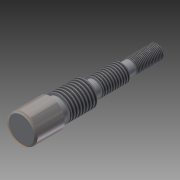
# Autodesk Inventor part: 13_3
Saved by Autodesk Inventor 2015 (Build 190159000, 159)
## iProperties
Created: 2015-03-30
Part Number: 13_3
Material: Generic
Document SubType Name: Modeling
Designer: WASHHSST
Density: 1 g/cm^3
Appearance: Default
Author: WASHHSST
Autodesk Inventor part; units mm, degrees
ref_plane "YZ Plane" through (0, 0, 0) normal (1, 0, 0) x (0, 1, 0)
ref_plane "XZ Plane" through (0, 0, 0) normal (0, 1, 0) x (-1, 0, 0)
ref_plane "XY Plane" through (0, 0, 0) normal (0, 0, 1) x (1, 0, 0)
sketch "Sketch2" plane through (0, 0, 0) normal (0, 0, 1) x (1, 0, 0)
  circle A0 centre (0, 0) radius 12.7
  dimension "d4" = 25.4
  constraints: 1 centre point, 1 coincident
  measures "d4" diameter of A0
extrude "Extrusion2" add sketch "Sketch2" against normal blind 25.4
chamfer "Chamfer1" distance 1.524 angle 45 1 edges at (-12.7, 0, 0) measured on face at (-12.2, 0, 0)
sketch "Sketch3" plane through (0, 0, -25.4) normal (0, 0, -1) x (-1, 0, 0)
  circle A0 centre (0, 0) radius 9.144
  dimension "d10" = 18.288
  constraints: 1 centre point, 1 coincident
  measures "d10" diameter of A0
extrude "Extrusion3" add sketch "Sketch3" along normal blind 6.35
sketch "Sketch4" plane through (0, 0, -31.75) normal (0, 0, -1) x (-1, 0, 0)
  circle A0 centre (0, 0) radius 11.049
  dimension "d13" = 22.098
  constraints: 1 centre point, 1 coincident
  measures "d13" diameter of A0
extrude "Extrusion4" add sketch "Sketch4" along normal blind 25.4
thread "Thread1" size "7/8-9 UNC" class "2A" standard "ANSI Unified Screw Threads" full length
chamfer "Chamfer2" distance 1.524 angle 45 1 edges at (11.049, 0, -57.15) measured on face at (10.549, 0, -57.15)
sketch "Sketch5" plane through (0, 0, -57.15) normal (0, 0, -1) x (-1, 0, 0)
  circle A0 centre (0, 0) radius 6.477
  dimension "d21" = 12.954
  constraints: 1 centre point, 1 coincident
  measures "d21" diameter of A0
extrude "Extrusion5" add sketch "Sketch5" along normal blind 6.35
sketch "Sketch6" plane through (0, 0, -63.5) normal (0, 0, -1) x (-1, 0, 0)
  circle A0 centre (0, 0) radius 7.874
  dimension "d24" = 15.748
  constraints: 1 centre point, 1 coincident
  measures "d24" diameter of A0
extrude "Extrusion6" add sketch "Sketch6" along normal blind 25.4
thread "Thread2" size "5/8-11 UNC" class "2A" standard "ANSI Unified Screw Threads" full length
chamfer "Chamfer3" distance 1.524 angle 45 1 edges at (7.874, 0, -88.9) measured on face at (7.374, 0, -88.9)
sketch "Sketch7" plane through (0, 0, -88.9) normal (0, 0, -1) x (-1, 0, 0)
  circle A0 centre (0, 0) radius 5.461
  dimension "d32" = 10.922
  constraints: 1 centre point, 1 coincident
  measures "d32" diameter of A0
extrude "Extrusion7" add sketch "Sketch7" along normal blind 6.35
sketch "Sketch8" plane through (0, 0, -95.25) normal (0, 0, -1) x (-1, 0, 0)
  circle A0 centre (0, 0) radius 6.35
  dimension "d35" = 12.7
  constraints: 1 centre point, 1 coincident
  measures "d35" diameter of A0
extrude "Extrusion8" add sketch "Sketch8" along normal blind 25.4
thread "Thread3" size "1/2-20 UNF" class "2A" standard "ANSI Unified Screw Threads" full length
chamfer "Chamfer4" distance 1.524 angle 45 1 edges at (6.35, 0, -120.65) measured on face at (5.85, 0, -120.65)
sketch "Sketch9" plane through (0, 0, 0) normal (0, 0, 1) x (1, 0, 0)
  circle A0 centre (0, 0) radius 12.7
  circle A1 centre (0, 0) radius 11.176 projected
  constraints: 1 centre point, 1 coincident, 1 concentric
surface extrude "ExtrusionSrf1" sketch "Sketch9" against normal blind 25.4 shown yes curves A0
body "Solid2"
body "Srf1"
